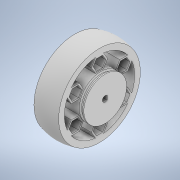
# Autodesk Inventor part: PulleyedWheelV1
Saved by Autodesk Inventor 2020 (Build 240168000, 168)
## iProperties
Created: 2023-12-21
Part Number: PulleyedWheelV1
Material: Generic
Document SubType Name: Modeling
Designer: smz3rm
Density: 1 g/cm^3
Appearance: Default
Author: smz3rm
Autodesk Inventor part; units mm, degrees
ref_plane "YZ Plane" through (0, 0, 0) normal (1, 0, 0) x (0, 1, 0)
ref_plane "XZ Plane" through (0, 0, 0) normal (0, 1, 0) x (-1, 0, 0)
ref_plane "XY Plane" through (0, 0, 0) normal (0, 0, 1) x (1, 0, 0)
sketch "Sketch1" plane through (0, 0, 0) normal (1, 0, 0) x (0, 1, 0)
  circle A0 centre (0, 0) radius 1.5
  line L0 (-25.2, 0) -> (25.2, 0) projected
  line L1 (1.118, -1) -> (-1.118, -1)
  circle A1 centre (0, 0) radius 11.25
  circle A2 centre (0, 0) radius 21.5
  circle A3 centre (0, 0) radius 18.5
  dimension "d0" = 3
  dimension "d1" = 1
  dimension "d3" = 43
  dimension "d4" = 3
  dimension "d6" = 22.5
  constraints: 4 centre point, 4 coincident, 2 end point, 2 point on circle, 1 horizontal
  measures "d0" diameter of A0
  measures "d1" distance between parallel lines of L0 L1
  measures "d3" diameter of A2
  measures "d4" radial gap between concentric circles of A2 A3
  measures "d6" diameter of A1
extrude "Extrusion1" add sketch "Sketch1" along normal blind 3 contours L1 A0 | A0 L0 A1 | L0 A1 A0
sketch "Sketch3" plane through (0, 0, 0) normal (0, 0, 1) x (1, 0, 0)
  line L0 (0, 11.25) -> (3, 11.25) projected
  line L1 (-0.6, 0) -> (3.6, 0) projected
  circle A0 centre (1.5, 10.75) radius 0.5
  line L2 (1.5, 10.75) -> (1.5, 11.25)
  line L3 (1.067, 10.5) -> (0.634, 11.25)
  line L4 (0, 11.25) -> (3, 11.25) projected
  line L5 (0, 10) -> (3, 10) projected
  line L6 (0, 11.25) -> (3, 11.25) projected
  line L7 (2.366, 11.25) -> (1.933, 10.5)
  point P0 (0, 0)
  dimension "d20" = 1
  dimension "d22" = 60
  dimension "d26" = 60
  constraints: 6 end point, 2 point on circle, 2 tangent, 1 centre point, 1 point on line, 1 vertical, 6 other
  measures "d20" diameter of A0
  measures "d22" angle to the sketch x axis of L3
  measures "d26" angle to the sketch x axis of L7
revolve "Revolution1" cut sketch "Sketch3" angle 360 about axis through (-10, 0, 0) along (1, 0, 0)
sketch "Sketch2" plane through (0, 0, 0) normal (-1, 0, 0) x (0, 0, 1)
  circle A0 centre (0, 0) radius 21.5
  circle A1 centre (0, 0) radius 18.5
  circle A2 centre (0, 0) radius 11.25 projected
  line L0 (-1, 1.118) -> (-1, -1.118) projected
  arc A3 (-1, -1.118) -> (-1, 1.118) centre (0, 0) ccw projected
  line L1 (2.1158, 18.3786) -> (4.2316, 14.7139)
  line L2 (4.2316, 14.7139) -> (2.1158, 11.0492)
  line L3 (2.1158, 11.0492) -> (-2.1158, 11.0492)
  line L4 (-2.1158, 11.0492) -> (-4.2316, 14.7139)
  line L5 (-4.2316, 14.7139) -> (-2.1158, 18.3786)
  line L6 (-2.1158, 18.3786) -> (2.1158, 18.3786)
  line L7 (0, -25.2) -> (0, 25.2) projected
  line L8 (-1.6539, 17.5786) -> (-3.3079, 14.7139)
  line L9 (-3.3079, 14.7139) -> (-1.6539, 11.8492)
  line L10 (-1.6539, 11.8492) -> (1.6539, 11.8492)
  line L11 (1.6539, 11.8492) -> (3.3079, 14.7139)
  line L12 (3.3079, 14.7139) -> (1.6539, 17.5786)
  line L13 (1.6539, 17.5786) -> (-1.6539, 17.5786)
  line L14 (-14.8584, 3.6923) -> (-16.9742, 7.357)
  line L15 (-10.6268, 3.6923) -> (-14.8584, 3.6923)
  line L16 (-8.511, 7.357) -> (-10.6268, 3.6923)
  line L17 (-16.9742, 7.357) -> (-14.8584, 11.0216)
  line L18 (-14.8584, 11.0216) -> (-10.6268, 11.0216)
  line L19 (-10.6268, 11.0216) -> (-8.511, 7.357)
  line L20 (-14.3966, 10.2216) -> (-16.0505, 7.357)
  line L21 (-16.0505, 7.357) -> (-14.3966, 4.4923)
  line L22 (-14.3966, 4.4923) -> (-11.0887, 4.4923)
  line L23 (-11.0887, 4.4923) -> (-9.4348, 7.357)
  line L24 (-9.4348, 7.357) -> (-11.0887, 10.2216)
  line L25 (-11.0887, 10.2216) -> (-14.3966, 10.2216)
  line L26 (-10.6268, -11.0216) -> (-14.8584, -11.0216)
  line L27 (-8.511, -7.357) -> (-10.6268, -11.0216)
  line L28 (-10.6268, -3.6923) -> (-8.511, -7.357)
  line L29 (-14.8584, -11.0216) -> (-16.9742, -7.357)
  line L30 (-16.9742, -7.357) -> (-14.8584, -3.6923)
  line L31 (-14.8584, -3.6923) -> (-10.6268, -3.6923)
  line L32 (-16.0505, -7.357) -> (-14.3966, -10.2216)
  line L33 (-14.3966, -10.2216) -> (-11.0887, -10.2216)
  line L34 (-11.0887, -10.2216) -> (-9.4348, -7.357)
  line L35 (-9.4348, -7.357) -> (-11.0887, -4.4923)
  line L36 (-11.0887, -4.4923) -> (-14.3966, -4.4923)
  line L37 (-14.3966, -4.4923) -> (-16.0505, -7.357)
  line L38 (4.2316, -14.7139) -> (2.1158, -18.3786)
  line L39 (2.1158, -11.0492) -> (4.2316, -14.7139)
  line L40 (-2.1158, -11.0492) -> (2.1158, -11.0492)
  line L41 (2.1158, -18.3786) -> (-2.1158, -18.3786)
  line L42 (-2.1158, -18.3786) -> (-4.2316, -14.7139)
  line L43 (-4.2316, -14.7139) -> (-2.1158, -11.0492)
  line L44 (-1.6539, -17.5786) -> (1.6539, -17.5786)
  line L45 (1.6539, -17.5786) -> (3.3079, -14.7139)
  line L46 (3.3079, -14.7139) -> (1.6539, -11.8492)
  line L47 (1.6539, -11.8492) -> (-1.6539, -11.8492)
  line L48 (-1.6539, -11.8492) -> (-3.3079, -14.7139)
  line L49 (-3.3079, -14.7139) -> (-1.6539, -17.5786)
  line L50 (14.8584, -3.6923) -> (16.9742, -7.357)
  line L51 (10.6268, -3.6923) -> (14.8584, -3.6923)
  line L52 (8.511, -7.357) -> (10.6268, -3.6923)
  line L53 (16.9742, -7.357) -> (14.8584, -11.0216)
  line L54 (14.8584, -11.0216) -> (10.6268, -11.0216)
  line L55 (10.6268, -11.0216) -> (8.511, -7.357)
  line L56 (14.3966, -10.2216) -> (16.0505, -7.357)
  line L57 (16.0505, -7.357) -> (14.3966, -4.4923)
  line L58 (14.3966, -4.4923) -> (11.0887, -4.4923)
  line L59 (11.0887, -4.4923) -> (9.4348, -7.357)
  line L60 (9.4348, -7.357) -> (11.0887, -10.2216)
  line L61 (11.0887, -10.2216) -> (14.3966, -10.2216)
  line L62 (10.6268, 11.0216) -> (14.8584, 11.0216)
  line L63 (8.511, 7.357) -> (10.6268, 11.0216)
  line L64 (10.6268, 3.6923) -> (8.511, 7.357)
  line L65 (14.8584, 11.0216) -> (16.9742, 7.357)
  line L66 (16.9742, 7.357) -> (14.8584, 3.6923)
  line L67 (14.8584, 3.6923) -> (10.6268, 3.6923)
  line L68 (16.0505, 7.357) -> (14.3966, 10.2216)
  line L69 (14.3966, 10.2216) -> (11.0887, 10.2216)
  line L70 (11.0887, 10.2216) -> (9.4348, 7.357)
  line L71 (9.4348, 7.357) -> (11.0887, 4.4923)
  line L72 (11.0887, 4.4923) -> (14.3966, 4.4923)
  line L73 (14.3966, 4.4923) -> (16.0505, 7.357)
  point P0 (0, 14.7139)
  point P1 (-2.1158, -18.3786)
  point P2 (-14.8584, -11.0216)
  point P3 (-8.511, -7.357)
  point P4 (-2.1158, -11.0492)
  point P5 (-8.511, 7.357)
  point P6 (-14.8584, 11.0216)
  point P7 (14.8584, 11.0216)
  point P8 (2.1158, 11.0492)
  point P9 (16.9742, -7.357)
  point P10 (10.6268, 3.6923)
  point P11 (16.9742, 7.357)
  point P12 (2.1158, -18.3786)
  point P13 (2.1158, -11.0492)
  point P14 (8.511, -7.357)
  point P15 (14.8584, -11.0216)
  point P16 (-10.6268, 3.6923)
  point P17 (-16.9742, -7.357)
  dimension "d9" = 43
  dimension "d10" = 3
  dimension "d11" = 0.8
  dimension "d14" = 360
  constraints: 144 end point, 2 centre point, 2 coincident, 2 point on circle, 1 point on line, 165 other
  measures "d9" diameter of A0
  measures "d10" radial gap between concentric circles of A0 A1
  measures "d11" distance between parallel lines of L5 L8
extrude "Extrusion2" add sketch "Sketch2" along normal blind 13 contours A0 L7 A1 | L7 A1 A0 | L7 L6 A1 | A1 L6 L7 | L7 L41 A1 | A1 L41 L7 | L1 L2 A2 L7 L10 L11 L12 L13 L6 | L6 L7 L13 L8 L9 L10 A2 L4 L5 | L42 L43 A2 L7 L47 L48 L49 L44 L41 | L41 L7 L44 L45 L46 L47 A2 L39 L38 | L65 L66 L67 A2 L63 L62 | A1 L65 | L17 A1 | L18 L19 A2 L15 L14 L17 | L29 L30 L31 A2 L27 L26 | A1 L29 | L53 A1 | L54 L55 A2 L51 L50 L53 | L3 L7 A2 | A2 L64 L52 L40 L7 A3 L3 | L3 L7 A3 L0 L40 A2 L28 L16 | A2 L7 L3 | L40 L7 A2 | A2 L7 L40 | A2 L64 | L16 A2 | A2 L28 | L52 A2
sketch "Sketch4" plane through (0, 0, 0) normal (0, 0, 1) x (1, 0, 0)
  line L0 (0, 21.5) -> (-13, 21.5) projected
  line L1 (-13, 21.5) -> (-13, -21.5) projected
  arc A0 (0, 21.5) -> (-13, 21.5) centre (-6.5, 0.875) ccw
  line L2 (-15.6, 0) -> (2.6, 0) projected
  point P0 (0, 0)
  point P1 (-6.5, 22.5)
  dimension "d24" = 1
  constraints: 3 point on circle, 1 centre point
  measures "d24" distance from line of L0 point (-6.5, 22.5)
revolve "Revolution2" add sketch "Sketch4" angle 360 about axis through (-10, 0, 0) along (1, 0, 0)
equation "\"d6\" = WheelGrooveDia"
equation "\"d7\" = WheelGrooveWidth"
equation "\"d20\" = WheelPulleyDia"
equation "\"d9\" = WheelDia - 2 * Roundedness"
equation "\"d16\" = WheelWidth"
equation "\"d24\" = Roundedness"
equation "\"Roundedness\" = 1"
equation "\"WheelGrooveDia\" = 22.5"
equation "\"WheelGrooveWidth\" = 3"
equation "\"WheelPulleyDia\" = 1"
equation "\"WheelDia\" = 45"
equation "\"WheelWidth\" = 13"
body "Solid1"
